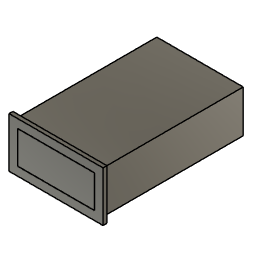
Auber 32 Din v2 (Autodesk Fusion 360 design; units mm, degrees)
Autodesk Fusion 360 part; units mm, degrees
sketch "Sketch1" plane through (0, 0, 0) normal (0, 0, 1) x (1, 0, 0)
  line L0 (0, 0) -> (45, 0)
  line L1 (45, 0) -> (45, 75)
  line L2 (45, 75) -> (0, 75)
  line L3 (0, 75) -> (0, 0)
  dimension "d1" = 45
  dimension "d2" = 75
  constraint horizontal L0
  constraint vertical L1
  constraint horizontal L2
  constraint vertical L3
  constraint coincident L0.start L3.end
  measures "d1" distance of L0.start L0.end
  measures "d2" distance of L0.start L2.end
extrude "Extrude1" add sketch "Sketch1" along normal blind 22 makes body 1
sketch "Sketch2" plane through (0, 0, 0) normal (0, -1, 0) x (1, 0, 0)
  line L0 (0, 0) -> (45, 0)
  line L1 (45, 0) -> (45, 22)
  line L2 (45, 22) -> (0, 22)
  line L3 (0, 22) -> (0, 0)
extrude "Extrude2" add sketch "Sketch2" against normal blind 2 separate body makes body 2
extrude "Extrude3" add 1 faces at (30, 0.6667, 22) along direction (0, 0, 1) blind 2 separate body on bodies 2 makes body 3
extrude "Extrude4" add 2 faces at (45, 0.6667, 22.6667) (45, 0.6667, 7.3333) along direction (1, 0, 0) blind 2 separate body on bodies 2 3 makes body 4
extrude "Extrude5" add 2 faces at (15, 0.6667, 0) (45.6667, 0.6667, 0) along direction (0, 0, -1) blind 2 separate body on bodies 2 4 makes body 5
extrude "Extrude6" add 3 faces at (0, 0.6667, 22.6667) (0, 0.6667, 14.6667) (0, 0.6667, -0.6667) along direction (-1, 0, 0) blind 2 on bodies 2 3 5 bodies 1 4 3 2 5
combine "Combine1" operation add target body 4 tool bodies 1
sketch "Sketch3" plane through (0, 0, 0) normal (0, -1, 0) x (1, 0, 0)
  line L0 (47, -2) -> (47, 24)
  line L1 (47, 24) -> (-2, 24)
  line L2 (-2, 24) -> (-2, -2)
  line L3 (-2, -2) -> (47, -2)
  line L4 (2.5, 2.5) -> (42.5, 2.5)
  line L5 (42.5, 2.5) -> (42.5, 19.5)
  line L6 (42.5, 19.5) -> (2.5, 19.5)
  line L7 (2.5, 19.5) -> (2.5, 2.5)
  dimension "d16" = 40
  dimension "d17" = 17
  constraint horizontal L4
  constraint vertical L5
  constraint horizontal L6
  constraint vertical L7
  measures "d16" distance of L4.start L4.end
  measures "d17" distance of L4.start L6.end
extrude "Extrude7" cut sketch "Sketch3" against normal blind 0.05 contours L4 L5 L6 L7 bodies 4
